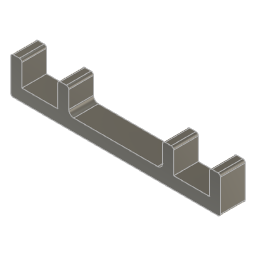
Link plate (Autodesk Fusion 360 design; units mm, degrees)
Autodesk Fusion 360 part; units mm, degrees
sketch "Sketch1" plane through (0, 0, 0) normal (0, 1, 0) x (1, 0, 0)
  line L0 (-1.75, -12) -> (5.5, -12)
  line L1 (5.5, -12) -> (5.5, -21)
  line L2 (6.5, -22) -> (9, -22)
  line L3 (10, -21) -> (10, -14)
  line L4 (29, -22) -> (29, -8.2498) construction
  line L5 (12, -12) -> (29, -12)
  line L6 (-1.75, -23.141) -> (-1.75, -10) construction
  arc A0 (5.5, -21) -> (6.5, -22) centre (6.5, -21) ccw
  arc A1 (9, -22) -> (10, -21) centre (9, -21) ccw
  line L7 (-1.75, -12) -> (-9, -12)
  line L8 (-9, -12) -> (-9, -21)
  arc A2 (-10, -22) -> (-9, -21) centre (-10, -21) ccw
  line L9 (-10, -22) -> (-12.5, -22)
  arc A3 (-13.5, -21) -> (-12.5, -22) centre (-12.5, -21) ccw
  line L10 (-13.5, -21) -> (-13.5, -12)
  line L11 (-13.5, -12) -> (-13.5, -8)
  line L12 (-12.5, -7) -> (29, -7)
  arc A4 (12, -12) -> (10, -14) centre (12, -14) ccw
  arc A5 (-12.5, -7) -> (-13.5, -8) centre (-12.5, -8) ccw
  line L13 (71.5, -12) -> (71.5, -8)
  arc A6 (51.5, -22) -> (52.5, -21) centre (51.5, -21) ccw
  arc A7 (48, -14) -> (46, -12) centre (46, -14) ccw
  line L14 (51.5, -22) -> (49, -22)
  arc A8 (67, -21) -> (68, -22) centre (68, -21) ccw
  line L15 (46, -12) -> (29, -12)
  line L16 (59.75, -12) -> (52.5, -12)
  line L17 (59.75, -12) -> (67, -12)
  line L18 (67, -12) -> (67, -21)
  arc A9 (70.5, -22) -> (71.5, -21) centre (70.5, -21) ccw
  line L19 (71.5, -21) -> (71.5, -12)
  arc A10 (48, -21) -> (49, -22) centre (49, -21) ccw
  line L20 (52.5, -12) -> (52.5, -21)
  line L21 (70.5, -7) -> (29, -7)
  line L22 (48, -21) -> (48, -14)
  line L23 (68, -22) -> (70.5, -22)
  arc A11 (71.5, -8) -> (70.5, -7) centre (70.5, -8) ccw
  point P0 (29, -8.2498)
  point P1 (59.75, -23.141)
  point P2 (29, -22)
  point P3 (59.75, -10)
  dimension "d1" = 1
  dimension "d4" = 2
  dimension "d5" = 1
  dimension "d8" = 19
  dimension "d10" = 4.5
  dimension "d11" = 15
  dimension "d12" = 5
  dimension "d13" = 7.25
  constraint horizontal L0
  constraint perpendicular L0 L1
  constraint perpendicular L1 L2
  constraint perpendicular L2 L3
  constraint vertical L4
  constraint coincident L4 L5.end
  constraint perpendicular L4 L5
  constraint perpendicular L0 L6
  constraint coincident L0.start L6
  constraint tangent L1 A0
  constraint tangent L2 A0
  constraint tangent L2 A1
  constraint tangent L3 A1
  constraint equal A0 A1
  constraint symmetric L0.start L6 L7.start
  constraint symmetric L0.end L6 L7.end
  constraint symmetric L6 L1.end L8.end
  constraint symmetric L6 L2.start A2.start
  constraint symmetric L6 A0 A2
  constraint symmetric L6 L2.end L9.end
  constraint symmetric L6 L3.start A3.start
  constraint symmetric L6 A1 A3
  constraint parallel L10 L11
  constraint perpendicular L10 L12
  constraint tangent L3 A4
  constraint tangent L5 A4
  constraint tangent L11 A5
  constraint tangent L12 A5
  constraint symmetric L0.start L4 L16.start
  constraint symmetric L0.end L4 L16.end
  constraint symmetric P2 L4 L4.start
  constraint symmetric P0 L4 L4.end
  constraint symmetric L4 L5.end L15.end
  constraint symmetric L4 L6.start P1
  constraint symmetric L4 L6.end P3
  constraint symmetric L4 L1.end A6.end
  constraint symmetric L4 L2.start A6.start
  constraint symmetric L4 A0 A6
  constraint symmetric L4 L2.end L14.end
  constraint symmetric L4 L3.start A10.start
  constraint symmetric L4 A1 A10
  constraint symmetric L4 L0.start L16.start
  constraint symmetric L4 L7.end L17.end
  constraint symmetric L4 L8.end A8.start
  constraint symmetric L4 A2.start A8.end
  constraint symmetric L4 A2 A8
  constraint symmetric L4 L9.end A9.start
  constraint symmetric L4 A3.start A9.end
  constraint symmetric L4 A3 A9
  constraint symmetric L4 L10.end L13.start
  constraint symmetric L4 L12.end L21.end
  constraint symmetric L4 L3.end A7.start
  constraint symmetric L4 L5.start A7.end
  constraint symmetric L4 A4 A7
  constraint symmetric L4 L11.end L13.end
  constraint symmetric L4 L12.start L21.start
  constraint symmetric L4 A5 A11
  measures "d1" radius of A0
  measures "d4" radius of A4
  measures "d5" radius of A5
  measures "d8" distance of L3 L4
  measures "d10" distance of L1 L3
  measures "d11" distance of L2 L12
  measures "d12" distance of L5 L12
  measures "d13" distance of L1 L6
extrude "Extrude1" add sketch "Sketch1" along normal blind 10
